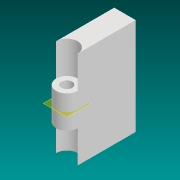
# Autodesk Inventor part: 连接块2
Saved by Autodesk Inventor 2021 (Build 250183000, 183)
## iProperties
Created: 2025-04-18
Part Number: 连接块2
Material: 常规
Document SubType Name: Modeling
Designer: 86155
Density: 1 g/cm^3
Appearance: 默认
Author: 86155
Autodesk Inventor part; units mm, degrees
ref_plane "YZ Plane" through (0, 0, 0) normal (1, 0, 0) x (0, 1, 0)
ref_plane "XZ Plane" through (0, 0, 0) normal (0, 1, 0) x (-1, 0, 0)
ref_plane "XY Plane" through (0, 0, 0) normal (0, 0, 1) x (1, 0, 0)
sketch "草图1" plane through (0, 0, 0) normal (0, 1, 0) x (-1, 0, 0)
  circle A0 centre (0, 0) radius 5
  circle A1 centre (0, 0) radius 2.5
  dimension "d0" = 10
  dimension "d1" = 5
  constraints: 2 centre point, 2 coincident
  measures "d0" diameter of A0
  measures "d1" diameter of A1
extrude "拉伸1" add sketch "草图1" along normal blind 15
ref_plane "工作平面1" through (0, 7.5, 0) normal (0, 1, 0) x (1, 0, 0)
sketch "草图2" plane through (0, 7.5, 0) normal (0, 1, 0) x (1, 0, 0)
  line L0 (-5, 7) -> (5, 7)
  line L1 (5, 7) -> (5, 27)
  line L2 (5, 27) -> (-5, 27)
  line L3 (-5, 27) -> (-5, 7)
  circle A0 centre (0, 0) radius 5
  circle A1 centre (0, 0) radius 5 projected
  line L4 (5, 0) -> (5, 7)
  circle A2 centre (0, 0) radius 5 projected
  line L5 (-5, 0) -> (-5, 7)
  dimension "d4" = 10
  dimension "d5" = 20
  dimension "d6" = 7
  dimension "d7" = 10
  dimension "d8" = 5
  constraints: 12 end point, 2 parallel, 1 centre point, 1 coincident, 1 horizontal, 1 horizontal alignment, 1 perpendicular, 1 point on circle, 1 tangent, 1 vertical, 1 other
  measures "d4" distance of L2.end L1.end
  measures "d5" distance of L1.end L0.end
  measures "d6" distance from line of L0 point (0, 0)
  measures "d7" diameter of A0
  measures "d8" distance from line of point (0, 0) L1
extrude "拉伸2" add sketch "草图2" along normal mid plane 45 contours L3 L2 L1 L0 | L0 L4 A0 L5
sketch "草图3" plane through (-5, -15, -27) normal (-1, 0, 0) x (0, 0, 1)
  line L0 (27, 0) -> (0, 0) projected
  line L1 (0, 0) -> (0, 45) projected
  point P0 (27, 15)
  point P1 (10, 22.5)
  dimension "d11" = 22.5
  dimension "d12" = 10
  measures "d11" distance from line of L0 point (10, 22.5)
  measures "d12" distance from line of L1 point (10, 22.5)
hole "孔1" at (-5, 7.5, -17) direction (1, 0, 0) diameter 8.376 depth 27.3 thread size "M10x1.5" designation "M10" class "6H" standard "GB Metric profile"
